Autodesk Inventor part; units mm, degrees
(part 6 of 7)
  line L1462 (-26.3463, 48.5084) -> (-12.9119, 48.5084)
  line L1463 (-12.9119, 52.5084) -> (-26.3463, 52.5084)
  line L1464 (-12.9119, 52.5084) -> (-26.3463, 52.5084)
  line L1465 (-26.3463, 48.5084) -> (-12.9119, 48.5084)
  line L1466 (-26.3463, 48.5084) -> (-12.9119, 48.5084)
  line L1467 (-26.3463, 48.5084) -> (-12.9119, 48.5084)
  arc A1650 (-12.9119, 48.5084) -> (-12.9119, 52.5084) centre (-12.9119, 50.5084) ccw
  arc A1651 (-46.3463, 52.5084) -> (-46.3463, 48.5084) centre (-46.3463, 50.5084) ccw
  arc A1652 (-52.9119, 48.5084) -> (-52.9119, 52.5084) centre (-52.9119, 50.5084) ccw
  arc A1653 (-46.3463, 52.5084) -> (-46.3463, 48.5084) centre (-46.3463, 50.5084) ccw
  arc A1654 (-46.3463, 52.5084) -> (-46.3463, 48.5084) centre (-46.3463, 50.5084) ccw
  arc A1655 (-46.3463, 52.5084) -> (-46.3463, 48.5084) centre (-46.3463, 50.5084) ccw
  arc A1656 (-46.3463, 52.5084) -> (-46.3463, 48.5084) centre (-46.3463, 50.5084) ccw
  arc A1657 (-46.3463, 52.5084) -> (-46.3463, 48.5084) centre (-46.3463, 50.5084) ccw
  arc A1658 (-52.9119, 48.5084) -> (-52.9119, 52.5084) centre (-52.9119, 50.5084) ccw
  arc A1659 (-52.9119, 48.5084) -> (-52.9119, 52.5084) centre (-52.9119, 50.5084) ccw
  arc A1660 (-52.9119, 48.5084) -> (-52.9119, 52.5084) centre (-52.9119, 50.5084) ccw
  arc A1661 (-52.9119, 48.5084) -> (-52.9119, 52.5084) centre (-52.9119, 50.5084) ccw
  line L1468 (-42.4124, 59.4654) -> (-55.8468, 59.4654)
  line L1469 (-55.8468, 55.4654) -> (-42.4124, 55.4654)
  line L1470 (-55.8468, 55.4654) -> (-42.4124, 55.4654)
  line L1471 (-55.8468, 55.4654) -> (-42.4124, 55.4654)
  line L1472 (-55.8468, 55.4654) -> (-42.4124, 55.4654)
  line L1473 (-55.8468, 55.4654) -> (-42.4124, 55.4654)
  line L1474 (-42.4124, 59.4654) -> (-55.8468, 59.4654)
  line L1475 (-42.4124, 59.4654) -> (-55.8468, 59.4654)
  line L1476 (-42.4124, 59.4654) -> (-55.8468, 59.4654)
  line L1477 (-42.4124, 59.4654) -> (-55.8468, 59.4654)
  arc A1662 (-86.3463, 52.5084) -> (-86.3463, 48.5084) centre (-86.3463, 50.5084) ccw
  arc A1663 (-86.3463, 52.5084) -> (-86.3463, 48.5084) centre (-86.3463, 50.5084) ccw
  arc A1664 (-86.3463, 52.5084) -> (-86.3463, 48.5084) centre (-86.3463, 50.5084) ccw
  arc A1665 (-92.9119, 48.5084) -> (-92.9119, 52.5084) centre (-92.9119, 50.5084) ccw
  line L1478 (-82.4124, 59.4654) -> (-95.8468, 59.4654)
  line L1479 (-95.8468, 55.4654) -> (-82.4124, 55.4654)
  line L1480 (-86.3463, 48.5084) -> (-72.9119, 48.5084)
  line L1481 (-86.3463, 48.5084) -> (-72.9119, 48.5084)
  line L1482 (-86.3463, 48.5084) -> (-72.9119, 48.5084)
  line L1483 (-72.9119, 52.5084) -> (-86.3463, 52.5084)
  line L1484 (-72.9119, 52.5084) -> (-86.3463, 52.5084)
  line L1485 (-72.9119, 52.5084) -> (-86.3463, 52.5084)
  arc A1666 (-75.8468, 59.4654) -> (-75.8468, 55.4654) centre (-75.8468, 57.4654) ccw
  arc A1667 (-75.8468, 59.4654) -> (-75.8468, 55.4654) centre (-75.8468, 57.4654) ccw
  arc A1668 (-75.8468, 59.4654) -> (-75.8468, 55.4654) centre (-75.8468, 57.4654) ccw
  arc A1669 (-75.8468, 59.4654) -> (-75.8468, 55.4654) centre (-75.8468, 57.4654) ccw
  arc A1670 (-82.4124, 55.4654) -> (-82.4124, 59.4654) centre (-82.4124, 57.4654) ccw
  line L1486 (-66.3463, 48.5084) -> (-52.9119, 48.5084)
  line L1487 (-52.9119, 52.5084) -> (-66.3463, 52.5084)
  line L1488 (-52.9119, 52.5084) -> (-66.3463, 52.5084)
  line L1489 (-66.3463, 48.5084) -> (-52.9119, 48.5084)
  line L1490 (-52.9119, 52.5084) -> (-66.3463, 52.5084)
  line L1491 (-52.9119, 52.5084) -> (-66.3463, 52.5084)
  line L1492 (-52.9119, 52.5084) -> (-66.3463, 52.5084)
  line L1493 (-66.3463, 48.5084) -> (-52.9119, 48.5084)
  line L1494 (-66.3463, 48.5084) -> (-52.9119, 48.5084)
  line L1495 (-66.3463, 48.5084) -> (-52.9119, 48.5084)
  line L1496 (-46.3463, 48.5084) -> (-32.9119, 48.5084)
  line L1497 (-32.9119, 52.5084) -> (-46.3463, 52.5084)
  line L1498 (-32.9119, 52.5084) -> (-46.3463, 52.5084)
  line L1499 (-46.3463, 48.5084) -> (-32.9119, 48.5084)
  line L1500 (-32.9119, 52.5084) -> (-46.3463, 52.5084)
  line L1501 (-32.9119, 52.5084) -> (-46.3463, 52.5084)
  line L1502 (-32.9119, 52.5084) -> (-46.3463, 52.5084)
  line L1503 (-46.3463, 48.5084) -> (-32.9119, 48.5084)
  line L1504 (-46.3463, 48.5084) -> (-32.9119, 48.5084)
  line L1505 (-46.3463, 48.5084) -> (-32.9119, 48.5084)
  line L1506 (-46.3463, 48.5084) -> (-32.9119, 48.5084)
  line L1507 (-32.9119, 52.5084) -> (-46.3463, 52.5084)
  arc A1671 (-55.8468, 59.4654) -> (-55.8468, 55.4654) centre (-55.8468, 57.4654) ccw
  arc A1672 (-55.8468, 59.4654) -> (-55.8468, 55.4654) centre (-55.8468, 57.4654) ccw
  arc A1673 (-55.8468, 59.4654) -> (-55.8468, 55.4654) centre (-55.8468, 57.4654) ccw
  arc A1674 (-62.4124, 55.4654) -> (-62.4124, 59.4654) centre (-62.4124, 57.4654) ccw
  arc A1675 (-55.8468, 59.4654) -> (-55.8468, 55.4654) centre (-55.8468, 57.4654) ccw
  arc A1676 (-55.8468, 59.4654) -> (-55.8468, 55.4654) centre (-55.8468, 57.4654) ccw
  arc A1677 (-55.8468, 59.4654) -> (-55.8468, 55.4654) centre (-55.8468, 57.4654) ccw
  arc A1678 (-55.8468, 59.4654) -> (-55.8468, 55.4654) centre (-55.8468, 57.4654) ccw
  arc A1679 (-62.4124, 55.4654) -> (-62.4124, 59.4654) centre (-62.4124, 57.4654) ccw
  arc A1680 (-62.4124, 55.4654) -> (-62.4124, 59.4654) centre (-62.4124, 57.4654) ccw
  arc A1681 (-66.3463, 52.5084) -> (-66.3463, 48.5084) centre (-66.3463, 50.5084) ccw
  arc A1682 (-72.9119, 48.5084) -> (-72.9119, 52.5084) centre (-72.9119, 50.5084) ccw
  arc A1683 (-66.3463, 52.5084) -> (-66.3463, 48.5084) centre (-66.3463, 50.5084) ccw
  line L1508 (-62.4124, 59.4654) -> (-75.8468, 59.4654)
  line L1509 (-75.8468, 55.4654) -> (-62.4124, 55.4654)
  arc A1684 (-72.9119, 48.5084) -> (-72.9119, 52.5084) centre (-72.9119, 50.5084) ccw
  line L1510 (-62.4124, 59.4654) -> (-75.8468, 59.4654)
  line L1511 (-75.8468, 55.4654) -> (-62.4124, 55.4654)
  arc A1685 (-66.3463, 52.5084) -> (-66.3463, 48.5084) centre (-66.3463, 50.5084) ccw
  arc A1686 (-66.3463, 52.5084) -> (-66.3463, 48.5084) centre (-66.3463, 50.5084) ccw
  arc A1687 (-66.3463, 52.5084) -> (-66.3463, 48.5084) centre (-66.3463, 50.5084) ccw
  line L1512 (-62.4124, 59.4654) -> (-75.8468, 59.4654)
  line L1513 (-75.8468, 55.4654) -> (-62.4124, 55.4654)
  arc A1688 (-72.9119, 48.5084) -> (-72.9119, 52.5084) centre (-72.9119, 50.5084) ccw
  arc A1689 (-106.3463, 52.5084) -> (-106.3463, 48.5084) centre (-106.3463, 50.5084) ccw
  arc A1690 (-95.8468, 59.4654) -> (-95.8468, 55.4654) centre (-95.8468, 57.4654) ccw
  line L1514 (-92.9119, 52.5084) -> (-106.3463, 52.5084)
  line L1515 (-106.3463, 48.5084) -> (-92.9119, 48.5084)
  arc A1691 (-35.8468, 59.4654) -> (-35.8468, 55.4654) centre (-35.8468, 57.4654) ccw
  arc A1692 (-35.8468, 59.4654) -> (-35.8468, 55.4654) centre (-35.8468, 57.4654) ccw
  arc A1693 (-35.8468, 59.4654) -> (-35.8468, 55.4654) centre (-35.8468, 57.4654) ccw
  arc A1694 (-42.4124, 55.4654) -> (-42.4124, 59.4654) centre (-42.4124, 57.4654) ccw
  arc A1695 (-42.4124, 55.4654) -> (-42.4124, 59.4654) centre (-42.4124, 57.4654) ccw
  arc A1696 (-35.8468, 59.4654) -> (-35.8468, 55.4654) centre (-35.8468, 57.4654) ccw
  arc A1697 (-35.8468, 59.4654) -> (-35.8468, 55.4654) centre (-35.8468, 57.4654) ccw
  arc A1698 (-35.8468, 59.4654) -> (-35.8468, 55.4654) centre (-35.8468, 57.4654) ccw
  arc A1699 (-35.8468, 59.4654) -> (-35.8468, 55.4654) centre (-35.8468, 57.4654) ccw
  arc A1700 (-35.8468, 59.4654) -> (-35.8468, 55.4654) centre (-35.8468, 57.4654) ccw
  arc A1701 (-35.8468, 59.4654) -> (-35.8468, 55.4654) centre (-35.8468, 57.4654) ccw
  arc A1702 (-42.4124, 55.4654) -> (-42.4124, 59.4654) centre (-42.4124, 57.4654) ccw
  arc A1703 (-42.4124, 55.4654) -> (-42.4124, 59.4654) centre (-42.4124, 57.4654) ccw
  arc A1704 (-42.4124, 55.4654) -> (-42.4124, 59.4654) centre (-42.4124, 57.4654) ccw
  arc A1705 (44.1532, 73.4654) -> (44.1532, 69.4654) centre (44.1532, 71.4654) ccw
  arc A1706 (44.1532, 73.4654) -> (44.1532, 69.4654) centre (44.1532, 71.4654) ccw
  arc A1707 (44.1532, 73.4654) -> (44.1532, 69.4654) centre (44.1532, 71.4654) ccw
  arc A1708 (44.1532, 73.4654) -> (44.1532, 69.4654) centre (44.1532, 71.4654) ccw
  arc A1709 (44.1532, 73.4654) -> (44.1532, 69.4654) centre (44.1532, 71.4654) ccw
  arc A1710 (44.1532, 73.4654) -> (44.1532, 69.4654) centre (44.1532, 71.4654) ccw
  arc A1711 (44.1532, 73.4654) -> (44.1532, 69.4654) centre (44.1532, 71.4654) ccw
  arc A1712 (33.6537, 66.5084) -> (33.6537, 62.5084) centre (33.6537, 64.5084) ccw
  arc A1713 (27.0881, 62.5084) -> (27.0881, 66.5084) centre (27.0881, 64.5084) ccw
  arc A1714 (27.0881, 62.5084) -> (27.0881, 66.5084) centre (27.0881, 64.5084) ccw
  arc A1715 (33.6537, 66.5084) -> (33.6537, 62.5084) centre (33.6537, 64.5084) ccw
  arc A1716 (27.0881, 62.5084) -> (27.0881, 66.5084) centre (27.0881, 64.5084) ccw
  arc A1717 (27.0881, 62.5084) -> (27.0881, 66.5084) centre (27.0881, 64.5084) ccw
  arc A1718 (27.0881, 62.5084) -> (27.0881, 66.5084) centre (27.0881, 64.5084) ccw
  arc A1719 (27.0881, 62.5084) -> (27.0881, 66.5084) centre (27.0881, 64.5084) ccw
  arc A1720 (33.6537, 66.5084) -> (33.6537, 62.5084) centre (33.6537, 64.5084) ccw
  arc A1721 (33.6537, 66.5084) -> (33.6537, 62.5084) centre (33.6537, 64.5084) ccw
  arc A1722 (33.6537, 66.5084) -> (33.6537, 62.5084) centre (33.6537, 64.5084) ccw
  line L1516 (24.1532, 69.4654) -> (37.5876, 69.4654)
  line L1517 (37.5876, 73.4654) -> (24.1532, 73.4654)
  line L1518 (24.1532, 69.4654) -> (37.5876, 69.4654)
  line L1519 (24.1532, 69.4654) -> (37.5876, 69.4654)
  line L1520 (24.1532, 69.4654) -> (37.5876, 69.4654)
  line L1521 (24.1532, 69.4654) -> (37.5876, 69.4654)
  line L1522 (24.1532, 69.4654) -> (37.5876, 69.4654)
  line L1523 (37.5876, 73.4654) -> (24.1532, 73.4654)
  line L1524 (37.5876, 73.4654) -> (24.1532, 73.4654)
  line L1525 (37.5876, 73.4654) -> (24.1532, 73.4654)
  line L1526 (37.5876, 73.4654) -> (24.1532, 73.4654)
  line L1527 (37.5876, 73.4654) -> (24.1532, 73.4654)
  arc A1723 (37.5876, 69.4654) -> (37.5876, 73.4654) centre (37.5876, 71.4654) ccw
  arc A1724 (37.5876, 69.4654) -> (37.5876, 73.4654) centre (37.5876, 71.4654) ccw
  arc A1725 (37.5876, 69.4654) -> (37.5876, 73.4654) centre (37.5876, 71.4654) ccw
  arc A1726 (37.5876, 69.4654) -> (37.5876, 73.4654) centre (37.5876, 71.4654) ccw
  arc A1727 (37.5876, 69.4654) -> (37.5876, 73.4654) centre (37.5876, 71.4654) ccw
  arc A1728 (37.5876, 69.4654) -> (37.5876, 73.4654) centre (37.5876, 71.4654) ccw
  arc A1729 (44.1532, 73.4654) -> (44.1532, 69.4654) centre (44.1532, 71.4654) ccw
  arc A1730 (47.0881, 62.5084) -> (47.0881, 66.5084) centre (47.0881, 64.5084) ccw
  arc A1731 (47.0881, 62.5084) -> (47.0881, 66.5084) centre (47.0881, 64.5084) ccw
  arc A1732 (53.6537, 66.5084) -> (53.6537, 62.5084) centre (53.6537, 64.5084) ccw
  arc A1733 (47.0881, 62.5084) -> (47.0881, 66.5084) centre (47.0881, 64.5084) ccw
  arc A1734 (47.0881, 62.5084) -> (47.0881, 66.5084) centre (47.0881, 64.5084) ccw
  arc A1735 (47.0881, 62.5084) -> (47.0881, 66.5084) centre (47.0881, 64.5084) ccw
  arc A1736 (53.6537, 66.5084) -> (53.6537, 62.5084) centre (53.6537, 64.5084) ccw
  arc A1737 (53.6537, 66.5084) -> (53.6537, 62.5084) centre (53.6537, 64.5084) ccw
  line L1528 (57.5876, 73.4654) -> (44.1532, 73.4654)
  line L1529 (44.1532, 69.4654) -> (57.5876, 69.4654)
  line L1530 (57.5876, 73.4654) -> (44.1532, 73.4654)
  line L1531 (44.1532, 69.4654) -> (57.5876, 69.4654)
  line L1532 (44.1532, 69.4654) -> (57.5876, 69.4654)
  line L1533 (44.1532, 69.4654) -> (57.5876, 69.4654)
  line L1534 (44.1532, 69.4654) -> (57.5876, 69.4654)
  line L1535 (57.5876, 73.4654) -> (44.1532, 73.4654)
  line L1536 (57.5876, 73.4654) -> (44.1532, 73.4654)
  line L1537 (57.5876, 73.4654) -> (44.1532, 73.4654)
  arc A1738 (57.5876, 69.4654) -> (57.5876, 73.4654) centre (57.5876, 71.4654) ccw
  arc A1739 (64.1532, 73.4654) -> (64.1532, 69.4654) centre (64.1532, 71.4654) ccw
  line L1538 (53.6537, 62.5084) -> (67.0881, 62.5084)
  line L1539 (53.6537, 62.5084) -> (67.0881, 62.5084)
  line L1540 (53.6537, 62.5084) -> (67.0881, 62.5084)
  line L1541 (67.0881, 66.5084) -> (53.6537, 66.5084)
  line L1542 (67.0881, 66.5084) -> (53.6537, 66.5084)
  line L1543 (67.0881, 66.5084) -> (53.6537, 66.5084)
  arc A1740 (64.1532, 73.4654) -> (64.1532, 69.4654) centre (64.1532, 71.4654) ccw
  arc A1741 (64.1532, 73.4654) -> (64.1532, 69.4654) centre (64.1532, 71.4654) ccw
  arc A1742 (64.1532, 73.4654) -> (64.1532, 69.4654) centre (64.1532, 71.4654) ccw
  arc A1743 (64.1532, 73.4654) -> (64.1532, 69.4654) centre (64.1532, 71.4654) ccw
  arc A1744 (57.5876, 69.4654) -> (57.5876, 73.4654) centre (57.5876, 71.4654) ccw
  arc A1745 (57.5876, 69.4654) -> (57.5876, 73.4654) centre (57.5876, 71.4654) ccw
  arc A1746 (57.5876, 69.4654) -> (57.5876, 73.4654) centre (57.5876, 71.4654) ccw
  arc A1747 (57.5876, 69.4654) -> (57.5876, 73.4654) centre (57.5876, 71.4654) ccw
  arc A1748 (67.0881, 62.5084) -> (67.0881, 66.5084) centre (67.0881, 64.5084) ccw
  arc A1749 (67.0881, 62.5084) -> (67.0881, 66.5084) centre (67.0881, 64.5084) ccw
  arc A1750 (67.0881, 62.5084) -> (67.0881, 66.5084) centre (67.0881, 64.5084) ccw
  line L1544 (77.5876, 73.4654) -> (64.1532, 73.4654)
  line L1545 (77.5876, 73.4654) -> (64.1532, 73.4654)
  line L1546 (77.5876, 73.4654) -> (64.1532, 73.4654)
  line L1547 (64.1532, 69.4654) -> (77.5876, 69.4654)
  line L1548 (64.1532, 69.4654) -> (77.5876, 69.4654)
  line L1549 (64.1532, 69.4654) -> (77.5876, 69.4654)
  arc A1751 (73.6537, 66.5084) -> (73.6537, 62.5084) centre (73.6537, 64.5084) ccw
  arc A1752 (77.5876, 69.4654) -> (77.5876, 73.4654) centre (77.5876, 71.4654) ccw
  arc A1753 (77.5876, 69.4654) -> (77.5876, 73.4654) centre (77.5876, 71.4654) ccw
  arc A1754 (77.5876, 69.4654) -> (77.5876, 73.4654) centre (77.5876, 71.4654) ccw
  arc A1755 (84.1532, 73.4654) -> (84.1532, 69.4654) centre (84.1532, 71.4654) ccw
  arc A1756 (84.1532, 73.4654) -> (84.1532, 69.4654) centre (84.1532, 71.4654) ccw
  line L1550 (87.0881, 66.5084) -> (73.6537, 66.5084)
  arc A1757 (87.0881, 62.5084) -> (87.0881, 66.5084) centre (87.0881, 64.5084) ccw
  line L1551 (73.6537, 62.5084) -> (87.0881, 62.5084)
  line L1552 (84.1532, 69.4654) -> (97.5876, 69.4654)
  line L1553 (97.5876, 73.4654) -> (84.1532, 73.4654)
  arc A1758 (97.5876, 69.4654) -> (97.5876, 73.4654) centre (97.5876, 71.4654) ccw
  line L1554 (33.6537, 62.5084) -> (47.0881, 62.5084)
  line L1555 (47.0881, 66.5084) -> (33.6537, 66.5084)
  line L1556 (33.6537, 62.5084) -> (47.0881, 62.5084)
  line L1557 (47.0881, 66.5084) -> (33.6537, 66.5084)
  line L1558 (47.0881, 66.5084) -> (33.6537, 66.5084)
  line L1559 (47.0881, 66.5084) -> (33.6537, 66.5084)
  line L1560 (47.0881, 66.5084) -> (33.6537, 66.5084)
  line L1561 (33.6537, 62.5084) -> (47.0881, 62.5084)
  line L1562 (33.6537, 62.5084) -> (47.0881, 62.5084)
  line L1563 (33.6537, 62.5084) -> (47.0881, 62.5084)
  arc A1759 (13.6537, 66.5084) -> (13.6537, 62.5084) centre (13.6537, 64.5084) ccw
  arc A1760 (13.6537, 66.5084) -> (13.6537, 62.5084) centre (13.6537, 64.5084) ccw
  arc A1761 (13.6537, 66.5084) -> (13.6537, 62.5084) centre (13.6537, 64.5084) ccw
  arc A1762 (13.6537, 66.5084) -> (13.6537, 62.5084) centre (13.6537, 64.5084) ccw
  arc A1763 (13.6537, 66.5084) -> (13.6537, 62.5084) centre (13.6537, 64.5084) ccw
  arc A1764 (13.6537, 66.5084) -> (13.6537, 62.5084) centre (13.6537, 64.5084) ccw
  arc A1765 (7.0881, 62.5084) -> (7.0881, 66.5084) centre (7.0881, 64.5084) ccw
  arc A1766 (7.0881, 62.5084) -> (7.0881, 66.5084) centre (7.0881, 64.5084) ccw
  arc A1767 (7.0881, 62.5084) -> (7.0881, 66.5084) centre (7.0881, 64.5084) ccw
  arc A1768 (7.0881, 62.5084) -> (7.0881, 66.5084) centre (7.0881, 64.5084) ccw
  arc A1769 (17.5876, 69.4654) -> (17.5876, 73.4654) centre (17.5876, 71.4654) ccw
  arc A1770 (17.5876, 69.4654) -> (17.5876, 73.4654) centre (17.5876, 71.4654) ccw
  arc A1771 (17.5876, 69.4654) -> (17.5876, 73.4654) centre (17.5876, 71.4654) ccw
  arc A1772 (17.5876, 69.4654) -> (17.5876, 73.4654) centre (17.5876, 71.4654) ccw
  arc A1773 (17.5876, 69.4654) -> (17.5876, 73.4654) centre (17.5876, 71.4654) ccw
  arc A1774 (17.5876, 69.4654) -> (17.5876, 73.4654) centre (17.5876, 71.4654) ccw
  arc A1775 (24.1532, 73.4654) -> (24.1532, 69.4654) centre (24.1532, 71.4654) ccw
  arc A1776 (24.1532, 73.4654) -> (24.1532, 69.4654) centre (24.1532, 71.4654) ccw
  arc A1777 (24.1532, 73.4654) -> (24.1532, 69.4654) centre (24.1532, 71.4654) ccw
  arc A1778 (24.1532, 73.4654) -> (24.1532, 69.4654) centre (24.1532, 71.4654) ccw
  arc A1779 (24.1532, 73.4654) -> (24.1532, 69.4654) centre (24.1532, 71.4654) ccw
  arc A1780 (24.1532, 73.4654) -> (24.1532, 69.4654) centre (24.1532, 71.4654) ccw
  arc A1781 (24.1532, 73.4654) -> (24.1532, 69.4654) centre (24.1532, 71.4654) ccw
  arc A1782 (24.1532, 73.4654) -> (24.1532, 69.4654) centre (24.1532, 71.4654) ccw
  arc A1783 (24.1532, 73.4654) -> (24.1532, 69.4654) centre (24.1532, 71.4654) ccw
  arc A1784 (4.1532, 73.4654) -> (4.1532, 69.4654) centre (4.1532, 71.4654) ccw
  arc A1785 (4.1532, 73.4654) -> (4.1532, 69.4654) centre (4.1532, 71.4654) ccw
  arc A1786 (4.1532, 73.4654) -> (4.1532, 69.4654) centre (4.1532, 71.4654) ccw
  arc A1787 (4.1532, 73.4654) -> (4.1532, 69.4654) centre (4.1532, 71.4654) ccw
  arc A1788 (4.1532, 73.4654) -> (4.1532, 69.4654) centre (4.1532, 71.4654) ccw
  arc A1789 (4.1532, 73.4654) -> (4.1532, 69.4654) centre (4.1532, 71.4654) ccw
  arc A1790 (4.1532, 73.4654) -> (4.1532, 69.4654) centre (4.1532, 71.4654) ccw
  arc A1791 (4.1532, 73.4654) -> (4.1532, 69.4654) centre (4.1532, 71.4654) ccw
  arc A1792 (4.1532, 73.4654) -> (4.1532, 69.4654) centre (4.1532, 71.4654) ccw
  arc A1793 (-2.4124, 69.4654) -> (-2.4124, 73.4654) centre (-2.4124, 71.4654) ccw
  arc A1794 (-2.4124, 69.4654) -> (-2.4124, 73.4654) centre (-2.4124, 71.4654) ccw
  arc A1795 (-2.4124, 69.4654) -> (-2.4124, 73.4654) centre (-2.4124, 71.4654) ccw
  arc A1796 (-2.4124, 69.4654) -> (-2.4124, 73.4654) centre (-2.4124, 71.4654) ccw
  arc A1797 (-32.9119, 62.5084) -> (-32.9119, 66.5084) centre (-32.9119, 64.5084) ccw
  arc A1798 (-32.9119, 62.5084) -> (-32.9119, 66.5084) centre (-32.9119, 64.5084) ccw
  arc A1799 (-32.9119, 62.5084) -> (-32.9119, 66.5084) centre (-32.9119, 64.5084) ccw
  arc A1800 (-32.9119, 62.5084) -> (-32.9119, 66.5084) centre (-32.9119, 64.5084) ccw
  arc A1801 (-32.9119, 62.5084) -> (-32.9119, 66.5084) centre (-32.9119, 64.5084) ccw
  arc A1802 (-32.9119, 62.5084) -> (-32.9119, 66.5084) centre (-32.9119, 64.5084) ccw
  line L1564 (27.0881, 66.5084) -> (13.6537, 66.5084)
  line L1565 (13.6537, 62.5084) -> (27.0881, 62.5084)
  line L1566 (27.0881, 66.5084) -> (13.6537, 66.5084)
  line L1567 (13.6537, 62.5084) -> (27.0881, 62.5084)
  line L1568 (13.6537, 62.5084) -> (27.0881, 62.5084)
  line L1569 (27.0881, 66.5084) -> (13.6537, 66.5084)
  line L1570 (27.0881, 66.5084) -> (13.6537, 66.5084)
  line L1571 (27.0881, 66.5084) -> (13.6537, 66.5084)
  line L1572 (13.6537, 62.5084) -> (27.0881, 62.5084)
  line L1573 (13.6537, 62.5084) -> (27.0881, 62.5084)
  line L1574 (13.6537, 62.5084) -> (27.0881, 62.5084)
  line L1575 (27.0881, 66.5084) -> (13.6537, 66.5084)
  line L1576 (4.1532, 69.4654) -> (17.5876, 69.4654)
  line L1577 (4.1532, 69.4654) -> (17.5876, 69.4654)
  line L1578 (4.1532, 69.4654) -> (17.5876, 69.4654)
  line L1579 (4.1532, 69.4654) -> (17.5876, 69.4654)
  line L1580 (4.1532, 69.4654) -> (17.5876, 69.4654)
  line L1581 (4.1532, 69.4654) -> (17.5876, 69.4654)
  line L1582 (17.5876, 73.4654) -> (4.1532, 73.4654)
  line L1583 (17.5876, 73.4654) -> (4.1532, 73.4654)
  line L1584 (17.5876, 73.4654) -> (4.1532, 73.4654)
  line L1585 (17.5876, 73.4654) -> (4.1532, 73.4654)
  line L1586 (17.5876, 73.4654) -> (4.1532, 73.4654)
  line L1587 (17.5876, 73.4654) -> (4.1532, 73.4654)
  arc A1803 (7.0881, 62.5084) -> (7.0881, 66.5084) centre (7.0881, 64.5084) ccw
  arc A1804 (7.0881, 62.5084) -> (7.0881, 66.5084) centre (7.0881, 64.5084) ccw
  line L1588 (-6.3463, 62.5084) -> (7.0881, 62.5084)
  line L1589 (7.0881, 66.5084) -> (-6.3463, 66.5084)
  line L1590 (7.0881, 66.5084) -> (-6.3463, 66.5084)
  line L1591 (-6.3463, 62.5084) -> (7.0881, 62.5084)
  line L1592 (-6.3463, 62.5084) -> (7.0881, 62.5084)
  line L1593 (7.0881, 66.5084) -> (-6.3463, 66.5084)
  line L1594 (7.0881, 66.5084) -> (-6.3463, 66.5084)
  line L1595 (7.0881, 66.5084) -> (-6.3463, 66.5084)
  line L1596 (-6.3463, 62.5084) -> (7.0881, 62.5084)
  line L1597 (-6.3463, 62.5084) -> (7.0881, 62.5084)
  line L1598 (-6.3463, 62.5084) -> (7.0881, 62.5084)
  line L1599 (7.0881, 66.5084) -> (-6.3463, 66.5084)
  arc A1805 (-6.3463, 66.5084) -> (-6.3463, 62.5084) centre (-6.3463, 64.5084) ccw
  arc A1806 (-6.3463, 66.5084) -> (-6.3463, 62.5084) centre (-6.3463, 64.5084) ccw
  arc A1807 (-6.3463, 66.5084) -> (-6.3463, 62.5084) centre (-6.3463, 64.5084) ccw
  arc A1808 (-6.3463, 66.5084) -> (-6.3463, 62.5084) centre (-6.3463, 64.5084) ccw
  arc A1809 (-6.3463, 66.5084) -> (-6.3463, 62.5084) centre (-6.3463, 64.5084) ccw
  arc A1810 (-6.3463, 66.5084) -> (-6.3463, 62.5084) centre (-6.3463, 64.5084) ccw
  arc A1811 (-12.9119, 62.5084) -> (-12.9119, 66.5084) centre (-12.9119, 64.5084) ccw
  arc A1812 (-12.9119, 62.5084) -> (-12.9119, 66.5084) centre (-12.9119, 64.5084) ccw
  arc A1813 (-12.9119, 62.5084) -> (-12.9119, 66.5084) centre (-12.9119, 64.5084) ccw
  arc A1814 (-12.9119, 62.5084) -> (-12.9119, 66.5084) centre (-12.9119, 64.5084) ccw
  arc A1815 (-12.9119, 62.5084) -> (-12.9119, 66.5084) centre (-12.9119, 64.5084) ccw
  line L1600 (-2.4124, 73.4654) -> (-15.8468, 73.4654)
  line L1601 (-15.8468, 69.4654) -> (-2.4124, 69.4654)
  line L1602 (-2.4124, 73.4654) -> (-15.8468, 73.4654)
  line L1603 (-15.8468, 69.4654) -> (-2.4124, 69.4654)
  line L1604 (-2.4124, 73.4654) -> (-15.8468, 73.4654)
  line L1605 (-15.8468, 69.4654) -> (-2.4124, 69.4654)
  line L1606 (-2.4124, 73.4654) -> (-15.8468, 73.4654)
  line L1607 (-15.8468, 69.4654) -> (-2.4124, 69.4654)
  line L1608 (-2.4124, 73.4654) -> (-15.8468, 73.4654)
  line L1609 (-15.8468, 69.4654) -> (-2.4124, 69.4654)
  line L1610 (-15.8468, 69.4654) -> (-2.4124, 69.4654)
  line L1611 (-2.4124, 73.4654) -> (-15.8468, 73.4654)
  arc A1816 (-2.4124, 69.4654) -> (-2.4124, 73.4654) centre (-2.4124, 71.4654) ccw
  arc A1817 (-2.4124, 69.4654) -> (-2.4124, 73.4654) centre (-2.4124, 71.4654) ccw
  arc A1818 (-15.8468, 73.4654) -> (-15.8468, 69.4654) centre (-15.8468, 71.4654) ccw
  arc A1819 (-15.8468, 73.4654) -> (-15.8468, 69.4654) centre (-15.8468, 71.4654) ccw
  arc A1820 (-15.8468, 73.4654) -> (-15.8468, 69.4654) centre (-15.8468, 71.4654) ccw
  arc A1821 (-15.8468, 73.4654) -> (-15.8468, 69.4654) centre (-15.8468, 71.4654) ccw
  arc A1822 (-15.8468, 73.4654) -> (-15.8468, 69.4654) centre (-15.8468, 71.4654) ccw
  arc A1823 (-22.4124, 69.4654) -> (-22.4124, 73.4654) centre (-22.4124, 71.4654) ccw
  arc A1824 (-22.4124, 69.4654) -> (-22.4124, 73.4654) centre (-22.4124, 71.4654) ccw
  arc A1825 (-15.8468, 73.4654) -> (-15.8468, 69.4654) centre (-15.8468, 71.4654) ccw
  arc A1826 (-15.8468, 73.4654) -> (-15.8468, 69.4654) centre (-15.8468, 71.4654) ccw
  arc A1827 (-22.4124, 69.4654) -> (-22.4124, 73.4654) centre (-22.4124, 71.4654) ccw
  arc A1828 (-15.8468, 73.4654) -> (-15.8468, 69.4654) centre (-15.8468, 71.4654) ccw
  arc A1829 (-15.8468, 73.4654) -> (-15.8468, 69.4654) centre (-15.8468, 71.4654) ccw
  arc A1830 (-22.4124, 69.4654) -> (-22.4124, 73.4654) centre (-22.4124, 71.4654) ccw
  arc A1831 (-22.4124, 69.4654) -> (-22.4124, 73.4654) centre (-22.4124, 71.4654) ccw
  arc A1832 (-22.4124, 69.4654) -> (-22.4124, 73.4654) centre (-22.4124, 71.4654) ccw
  arc A1833 (-26.3463, 66.5084) -> (-26.3463, 62.5084) centre (-26.3463, 64.5084) ccw
  arc A1834 (-26.3463, 66.5084) -> (-26.3463, 62.5084) centre (-26.3463, 64.5084) ccw
  arc A1835 (-26.3463, 66.5084) -> (-26.3463, 62.5084) centre (-26.3463, 64.5084) ccw
  arc A1836 (-26.3463, 66.5084) -> (-26.3463, 62.5084) centre (-26.3463, 64.5084) ccw
  arc A1837 (-26.3463, 66.5084) -> (-26.3463, 62.5084) centre (-26.3463, 64.5084) ccw
  arc A1838 (-26.3463, 66.5084) -> (-26.3463, 62.5084) centre (-26.3463, 64.5084) ccw
  line L1612 (-35.8468, 69.4654) -> (-22.4124, 69.4654)
  line L1613 (-35.8468, 69.4654) -> (-22.4124, 69.4654)
  line L1614 (-35.8468, 69.4654) -> (-22.4124, 69.4654)
  line L1615 (-35.8468, 69.4654) -> (-22.4124, 69.4654)
  line L1616 (-35.8468, 69.4654) -> (-22.4124, 69.4654)
  line L1617 (-35.8468, 69.4654) -> (-22.4124, 69.4654)
  line L1618 (-22.4124, 73.4654) -> (-35.8468, 73.4654)
  line L1619 (-22.4124, 73.4654) -> (-35.8468, 73.4654)
  line L1620 (-22.4124, 73.4654) -> (-35.8468, 73.4654)
  line L1621 (-22.4124, 73.4654) -> (-35.8468, 73.4654)
  line L1622 (-22.4124, 73.4654) -> (-35.8468, 73.4654)
  line L1623 (-22.4124, 73.4654) -> (-35.8468, 73.4654)
  line L1624 (-26.3463, 62.5084) -> (-12.9119, 62.5084)
  line L1625 (-12.9119, 66.5084) -> (-26.3463, 66.5084)
  line L1626 (-12.9119, 66.5084) -> (-26.3463, 66.5084)
  line L1627 (-26.3463, 62.5084) -> (-12.9119, 62.5084)
  line L1628 (-12.9119, 66.5084) -> (-26.3463, 66.5084)
  line L1629 (-12.9119, 66.5084) -> (-26.3463, 66.5084)
  line L1630 (-26.3463, 62.5084) -> (-12.9119, 62.5084)
  line L1631 (-12.9119, 66.5084) -> (-26.3463, 66.5084)
  line L1632 (-12.9119, 66.5084) -> (-26.3463, 66.5084)
  line L1633 (-26.3463, 62.5084) -> (-12.9119, 62.5084)
  line L1634 (-26.3463, 62.5084) -> (-12.9119, 62.5084)
  line L1635 (-26.3463, 62.5084) -> (-12.9119, 62.5084)
  arc A1839 (-12.9119, 62.5084) -> (-12.9119, 66.5084) centre (-12.9119, 64.5084) ccw
  arc A1840 (-46.3463, 66.5084) -> (-46.3463, 62.5084) centre (-46.3463, 64.5084) ccw
  arc A1841 (-52.9119, 62.5084) -> (-52.9119, 66.5084) centre (-52.9119, 64.5084) ccw
  arc A1842 (-46.3463, 66.5084) -> (-46.3463, 62.5084) centre (-46.3463, 64.5084) ccw
  arc A1843 (-46.3463, 66.5084) -> (-46.3463, 62.5084) centre (-46.3463, 64.5084) ccw
  arc A1844 (-46.3463, 66.5084) -> (-46.3463, 62.5084) centre (-46.3463, 64.5084) ccw
  arc A1845 (-46.3463, 66.5084) -> (-46.3463, 62.5084) centre (-46.3463, 64.5084) ccw
  arc A1846 (-46.3463, 66.5084) -> (-46.3463, 62.5084) centre (-46.3463, 64.5084) ccw
  arc A1847 (-52.9119, 62.5084) -> (-52.9119, 66.5084) centre (-52.9119, 64.5084) ccw
  arc A1848 (-52.9119, 62.5084) -> (-52.9119, 66.5084) centre (-52.9119, 64.5084) ccw
  arc A1849 (-52.9119, 62.5084) -> (-52.9119, 66.5084) centre (-52.9119, 64.5084) ccw
  arc A1850 (-52.9119, 62.5084) -> (-52.9119, 66.5084) centre (-52.9119, 64.5084) ccw
  line L1636 (-42.4124, 73.4654) -> (-55.8468, 73.4654)
  line L1637 (-55.8468, 69.4654) -> (-42.4124, 69.4654)
  line L1638 (-55.8468, 69.4654) -> (-42.4124, 69.4654)
  line L1639 (-55.8468, 69.4654) -> (-42.4124, 69.4654)
  line L1640 (-55.8468, 69.4654) -> (-42.4124, 69.4654)
  line L1641 (-55.8468, 69.4654) -> (-42.4124, 69.4654)
  line L1642 (-42.4124, 73.4654) -> (-55.8468, 73.4654)
  line L1643 (-42.4124, 73.4654) -> (-55.8468, 73.4654)
  line L1644 (-42.4124, 73.4654) -> (-55.8468, 73.4654)
  line L1645 (-42.4124, 73.4654) -> (-55.8468, 73.4654)
  arc A1851 (-86.3463, 66.5084) -> (-86.3463, 62.5084) centre (-86.3463, 64.5084) ccw
  arc A1852 (-86.3463, 66.5084) -> (-86.3463, 62.5084) centre (-86.3463, 64.5084) ccw
  arc A1853 (-86.3463, 66.5084) -> (-86.3463, 62.5084) centre (-86.3463, 64.5084) ccw
  arc A1854 (-92.9119, 62.5084) -> (-92.9119, 66.5084) centre (-92.9119, 64.5084) ccw
  line L1646 (-82.4124, 73.4654) -> (-95.8468, 73.4654)
  line L1647 (-95.8468, 69.4654) -> (-82.4124, 69.4654)
  line L1648 (-86.3463, 62.5084) -> (-72.9119, 62.5084)
  line L1649 (-86.3463, 62.5084) -> (-72.9119, 62.5084)
  line L1650 (-86.3463, 62.5084) -> (-72.9119, 62.5084)
  line L1651 (-72.9119, 66.5084) -> (-86.3463, 66.5084)
  line L1652 (-72.9119, 66.5084) -> (-86.3463, 66.5084)
  line L1653 (-72.9119, 66.5084) -> (-86.3463, 66.5084)
  arc A1855 (-75.8468, 73.4654) -> (-75.8468, 69.4654) centre (-75.8468, 71.4654) ccw
  arc A1856 (-75.8468, 73.4654) -> (-75.8468, 69.4654) centre (-75.8468, 71.4654) ccw
  arc A1857 (-75.8468, 73.4654) -> (-75.8468, 69.4654) centre (-75.8468, 71.4654) ccw
  arc A1858 (-75.8468, 73.4654) -> (-75.8468, 69.4654) centre (-75.8468, 71.4654) ccw
  arc A1859 (-82.4124, 69.4654) -> (-82.4124, 73.4654) centre (-82.4124, 71.4654) ccw
  line L1654 (-66.3463, 62.5084) -> (-52.9119, 62.5084)
  line L1655 (-52.9119, 66.5084) -> (-66.3463, 66.5084)
  line L1656 (-52.9119, 66.5084) -> (-66.3463, 66.5084)
  line L1657 (-66.3463, 62.5084) -> (-52.9119, 62.5084)
  line L1658 (-52.9119, 66.5084) -> (-66.3463, 66.5084)
  line L1659 (-52.9119, 66.5084) -> (-66.3463, 66.5084)
  line L1660 (-52.9119, 66.5084) -> (-66.3463, 66.5084)
  line L1661 (-66.3463, 62.5084) -> (-52.9119, 62.5084)
  line L1662 (-66.3463, 62.5084) -> (-52.9119, 62.5084)
  line L1663 (-66.3463, 62.5084) -> (-52.9119, 62.5084)
  line L1664 (-46.3463, 62.5084) -> (-32.9119, 62.5084)
  line L1665 (-32.9119, 66.5084) -> (-46.3463, 66.5084)
  line L1666 (-32.9119, 66.5084) -> (-46.3463, 66.5084)
  line L1667 (-46.3463, 62.5084) -> (-32.9119, 62.5084)
  line L1668 (-32.9119, 66.5084) -> (-46.3463, 66.5084)
  line L1669 (-32.9119, 66.5084) -> (-46.3463, 66.5084)
  line L1670 (-32.9119, 66.5084) -> (-46.3463, 66.5084)
  line L1671 (-46.3463, 62.5084) -> (-32.9119, 62.5084)
  line L1672 (-46.3463, 62.5084) -> (-32.9119, 62.5084)
  line L1673 (-46.3463, 62.5084) -> (-32.9119, 62.5084)
  line L1674 (-46.3463, 62.5084) -> (-32.9119, 62.5084)
  line L1675 (-32.9119, 66.5084) -> (-46.3463, 66.5084)
  arc A1860 (-55.8468, 73.4654) -> (-55.8468, 69.4654) centre (-55.8468, 71.4654) ccw
  arc A1861 (-55.8468, 73.4654) -> (-55.8468, 69.4654) centre (-55.8468, 71.4654) ccw
  arc A1862 (-55.8468, 73.4654) -> (-55.8468, 69.4654) centre (-55.8468, 71.4654) ccw
  arc A1863 (-62.4124, 69.4654) -> (-62.4124, 73.4654) centre (-62.4124, 71.4654) ccw
  arc A1864 (-55.8468, 73.4654) -> (-55.8468, 69.4654) centre (-55.8468, 71.4654) ccw
  arc A1865 (-55.8468, 73.4654) -> (-55.8468, 69.4654) centre (-55.8468, 71.4654) ccw
  arc A1866 (-55.8468, 73.4654) -> (-55.8468, 69.4654) centre (-55.8468, 71.4654) ccw
  arc A1867 (-55.8468, 73.4654) -> (-55.8468, 69.4654) centre (-55.8468, 71.4654) ccw
  arc A1868 (-62.4124, 69.4654) -> (-62.4124, 73.4654) centre (-62.4124, 71.4654) ccw
  arc A1869 (-62.4124, 69.4654) -> (-62.4124, 73.4654) centre (-62.4124, 71.4654) ccw
  arc A1870 (-66.3463, 66.5084) -> (-66.3463, 62.5084) centre (-66.3463, 64.5084) ccw
  arc A1871 (-72.9119, 62.5084) -> (-72.9119, 66.5084) centre (-72.9119, 64.5084) ccw
  arc A1872 (-66.3463, 66.5084) -> (-66.3463, 62.5084) centre (-66.3463, 64.5084) ccw
  line L1676 (-62.4124, 73.4654) -> (-75.8468, 73.4654)
  line L1677 (-75.8468, 69.4654) -> (-62.4124, 69.4654)
  arc A1873 (-72.9119, 62.5084) -> (-72.9119, 66.5084) centre (-72.9119, 64.5084) ccw
  line L1678 (-62.4124, 73.4654) -> (-75.8468, 73.4654)
  line L1679 (-75.8468, 69.4654) -> (-62.4124, 69.4654)
  arc A1874 (-66.3463, 66.5084) -> (-66.3463, 62.5084) centre (-66.3463, 64.5084) ccw
  arc A1875 (-66.3463, 66.5084) -> (-66.3463, 62.5084) centre (-66.3463, 64.5084) ccw
  arc A1876 (-66.3463, 66.5084) -> (-66.3463, 62.5084) centre (-66.3463, 64.5084) ccw
  line L1680 (-62.4124, 73.4654) -> (-75.8468, 73.4654)
  line L1681 (-75.8468, 69.4654) -> (-62.4124, 69.4654)
  arc A1877 (-72.9119, 62.5084) -> (-72.9119, 66.5084) centre (-72.9119, 64.5084) ccw
  arc A1878 (-106.3463, 66.5084) -> (-106.3463, 62.5084) centre (-106.3463, 64.5084) ccw
  arc A1879 (-95.8468, 73.4654) -> (-95.8468, 69.4654) centre (-95.8468, 71.4654) ccw
  line L1682 (-92.9119, 66.5084) -> (-106.3463, 66.5084)
  line L1683 (-106.3463, 62.5084) -> (-92.9119, 62.5084)
  arc A1880 (-35.8468, 73.4654) -> (-35.8468, 69.4654) centre (-35.8468, 71.4654) ccw
  arc A1881 (-35.8468, 73.4654) -> (-35.8468, 69.4654) centre (-35.8468, 71.4654) ccw
  arc A1882 (-35.8468, 73.4654) -> (-35.8468, 69.4654) centre (-35.8468, 71.4654) ccw
  arc A1883 (-42.4124, 69.4654) -> (-42.4124, 73.4654) centre (-42.4124, 71.4654) ccw
  arc A1884 (-42.4124, 69.4654) -> (-42.4124, 73.4654) centre (-42.4124, 71.4654) ccw
  arc A1885 (-35.8468, 73.4654) -> (-35.8468, 69.4654) centre (-35.8468, 71.4654) ccw
  arc A1886 (-35.8468, 73.4654) -> (-35.8468, 69.4654) centre (-35.8468, 71.4654) ccw
  arc A1887 (-35.8468, 73.4654) -> (-35.8468, 69.4654) centre (-35.8468, 71.4654) ccw
  arc A1888 (-35.8468, 73.4654) -> (-35.8468, 69.4654) centre (-35.8468, 71.4654) ccw
  arc A1889 (-35.8468, 73.4654) -> (-35.8468, 69.4654) centre (-35.8468, 71.4654) ccw
  arc A1890 (-35.8468, 73.4654) -> (-35.8468, 69.4654) centre (-35.8468, 71.4654) ccw
  arc A1891 (-42.4124, 69.4654) -> (-42.4124, 73.4654) centre (-42.4124, 71.4654) ccw
  arc A1892 (-42.4124, 69.4654) -> (-42.4124, 73.4654) centre (-42.4124, 71.4654) ccw
  arc A1893 (-42.4124, 69.4654) -> (-42.4124, 73.4654) centre (-42.4124, 71.4654) ccw
  line L1684 (-75, 70) -> (75, 70)
  line L1685 (85, 60) -> (85, -60)
  line L1686 (75, -70) -> (-75, -70)
  line L1687 (-85, -60) -> (-85, 60)
  line L1688 (85, 70) -> (-85, -70) construction
  line L1689 (-78, 73) -> (78, 73)
  line L1690 (88, 63) -> (88, -63)
  line L1691 (78, -73) -> (-78, -73)
  line L1692 (-88, -63) -> (-88, 63)
  line L1693 (-88, 73) -> (88, -73) construction
  arc A1894 (-75, 70) -> (-85, 60) centre (-75, 60) ccw
  arc A1895 (-78, 73) -> (-88, 63) centre (-78, 63) ccw
  arc A1896 (85, 60) -> (75, 70) centre (75, 60) ccw
  arc A1897 (88, 63) -> (78, 73) centre (78, 63) ccw
  arc A1898 (75, -70) -> (85, -60) centre (75, -60) ccw
  arc A1899 (78, -73) -> (88, -63) centre (78, -63) ccw
  arc A1900 (-88, -63) -> (-78, -73) centre (-78, -63) ccw
  arc A1901 (-85, -60) -> (-75, -70) centre (-75, -60) ccw
  circle A1902 centre (-73.7339, -61.8573) radius 1.25
  line L1694 (0, 0) -> (0, 1.4904)
  line L1695 (0, 0) -> (1.3651, 0)
  line L1696 (-73.7339, -52.8401) -> (-85, -52.8401)
  line L1697 (-64.7396, -62.5) -> (-64.7396, -70)
  arc A1903 (-64.7396, -62.5) -> (-74.5, -52.8727) centre (-73.7339, -61.8573) ccw
  arc A1904 (74.5, -52.8727) -> (64.7396, -62.5) centre (73.7339, -61.8573) ccw
  line L1698 (64.7396, -62.5) -> (64.7396, -70)
  line L1699 (73.7339, -52.8401) -> (85, -52.8401)
  circle A1905 centre (73.7339, -61.8573) radius 1.25
  line L1700 (-80, -42) -> (-77, -42)
  circle A1906 centre (-77, -42) radius 1.25
  arc A1907 (-69.0044, -42.2652) -> (-77, -34) centre (-77, -42) ccw
  line L1701 (-77, -34) -> (-85, -34)
  line L1702 (-69, -42) -> (-69, -54.1827)
  arc A1908 (77, -34) -> (69.0044, -42.2652) centre (77, -42) ccw
  line L1703 (69, -42) -> (69, -54.1827)
  circle A1909 centre (77, -42) radius 1.25
  line L1704 (-77, 34) -> (-85, 34)
  arc A1910 (-77, 34) -> (-69.0044, 42.2652) centre (-77, 42) ccw
  line L1705 (-69, 42) -> (-69, 54.1827)
  line L1706 (69, 42) -> (69, 54.1827)
  arc A1911 (69.0044, 42.2652) -> (77, 34) centre (77, 42) ccw
  line L1707 (77, -34) -> (85, -34)
  line L1708 (77, 34) -> (85, 34)
  line L1709 (64.7396, 62.5) -> (64.7396, 70)
  arc A1912 (64.7396, 62.5) -> (74.5, 52.8727) centre (73.7339, 61.8573) ccw
  line L1710 (73.7339, 52.8401) -> (85, 52.8401)
  circle A1913 centre (73.7339, 61.8573) radius 1.25
  line L1711 (-64.7396, 62.5) -> (-64.7396, 70)
  arc A1914 (-74.5, 52.8727) -> (-64.7396, 62.5) centre (-73.7339, 61.8573) ccw
  circle A1915 centre (-73.7339, 61.8573) radius 1.25
  line L1712 (-73.7339, 52.8401) -> (-85, 52.8401)
  circle A1916 centre (-73.7339, 61.8573) radius 1.25
  circle A1917 centre (73.7339, 61.8573) radius 1.25
  circle A1918 centre (77, 42) radius 1.25
  circle A1919 centre (-77, 42) radius 1.25
  point P0 (80, -38.5)
  point P1 (70, -38.5)
  point P2 (70, -48.5)
  point P3 (-70, -48.5)
  point P4 (-70, -38.5)
  point P5 (-80, -38.5)
  point P6 (80, -24.5)
  point P7 (70, -24.5)
  point P8 (70, -34.5)
  point P9 (-70, -34.5)
  point P10 (-70, -24.5)
  point P11 (-80, -24.5)
  point P12 (80, -10.5)
  point P13 (70, -10.5)
  point P14 (70, -20.5)
  point P15 (-70, -20.5)
  point P16 (-70, -10.5)
  point P17 (-80, -10.5)
  point P18 (80, 3.5)
  point P19 (70, 3.5)
  point P20 (70, -6.5)
  point P21 (-70, -6.5)
  point P22 (-70, 3.5)
  point P23 (-80, 3.5)
  point P24 (80, 17.5)
  point P25 (70, 17.5)
  point P26 (70, 7.5)
  point P27 (-70, 7.5)
  point P28 (-70, 17.5)
  point P29 (-80, 17.5)
  point P30 (80, 31.5)
  point P31 (70, 31.5)
  point P32 (70, 21.5)
  point P33 (-70, 21.5)
  point P34 (-70, 31.5)
  point P35 (-80, 31.5)
  point P36 (80, 45.5)
  point P37 (70, 45.5)
  point P38 (70, 35.5)
  point P39 (-70, 35.5)
  point P40 (-70, 45.5)
  point P41 (-80, 45.5)
  point P42 (80, 59.5)
  point P43 (70, 59.5)
  point P44 (70, 49.5)
  point P45 (-70, 49.5)
  point P46 (-70, 59.5)
  point P47 (-80, 59.5)
  point P48 (80, 73.5)
  point P49 (70, 73.5)
  point P50 (70, 63.5)
  point P51 (-70, 63.5)
  point P52 (-70, 73.5)
  point P53 (-80, 73.5)
  point P54 (80, -17.4916)
  point P55 (80, -7.4916)
  point P56 (80, -3.4916)
  point P57 (80, 6.5084)
  point P58 (80, 10.5084)
  point P59 (80, 20.5084)
  point P60 (80, 34)
  point P61 (74.1935, 34.5084)
  point P62 (71.7227, 35.9875)
  point P63 (69.0179, 41.4654)
  point P64 (69, 45.4654)
  point P65 (69, 49.9213)
  point P66 (69, 51.0956)
  point P67 (67.3736, 55.4654)
  point P68 (65.0397, 59.4654)
  point P69 (-65.0397, 59.4654)
  point P70 (-67.3736, 55.4654)
  point P71 (-69, 45.4654)
  point P72 (-69.0179, 41.4654)
  point P73 (-70.9314, 36.7873)
  point P74 (-74.1935, 34.5084)
  point P75 (-80, 34)
  point P76 (-80, 24.5084)
  point P77 (-80, 20.5084)
  point P78 (-80, 10.5084)
  point P79 (-80, 6.5084)
  point P80 (-80, -3.4916)
  point P81 (-80, -7.4916)
  point P82 (-80, -17.4916)
  point P83 (-80, -21.4916)
  point P84 (-80, -31.4916)
  point P85 (-72.4312, -35.433)
  point P86 (-69.7895, -38.5346)
  point P87 (-69, -42.5346)
  point P88 (-69, -52.5346)
  point P89 (-66.4553, -56.5346)
  point P90 (-65.0326, -59.4916)
  point P91 (-51.1847, -62.5)
  point P92 (-48.0735, -62.5)
  point P93 (-31.1847, -62.5)
  point P94 (-28.0735, -62.5)
  point P95 (-11.1847, -62.5)
  point P96 (-8.0735, -62.5)
  point P97 (8.8153, -62.5)
  point P98 (11.9265, -62.5)
  point P99 (28.8153, -62.5)
  point P100 (31.9265, -62.5)
  point P101 (48.8153, -62.5)
  point P102 (51.9265, -62.5)
  point P103 (65.0326, -59.4916)
  point P104 (66.4553, -56.5346)
  point P105 (69, -52.5346)
  point P106 (69, -48.0787)
  point P107 (69, -46.9044)
  point P108 (69, -42.5346)
  point P109 (69.7895, -38.5346)
  point P110 (72.7037, -35.2515)
  point P111 (80, -31.4916)
  point P112 (80, -21.4916)
  point P113 (-22.4124, 59.4654)
  point P114 (-2.4124, 59.4654)
  point P115 (-2.4124, 55.4654)
  point P116 (17.5876, 59.4654)
  point P117 (17.5876, 55.4654)
  point P118 (-22.4124, 45.4654)
  point P119 (-2.4124, 45.4654)
  point P120 (-2.4124, 41.4654)
  point P121 (17.5876, 45.4654)
  point P122 (17.5876, 41.4654)
  point P123 (44.1532, 41.4654)
  point P124 (44.1532, 27.4654)
  point P125 (53.6537, 10.5084)
  point P126 (44.1532, 13.4654)
  point P127 (53.6537, -3.4916)
  point P128 (44.1532, -0.5346)
  point P129 (53.6537, -17.4916)
  point P130 (44.1532, -14.5346)
  point P131 (64.1532, -28.5346)
  point P132 (-22.4124, -38.5346)
  point P133 (-2.4124, -38.5346)
  point P134 (-2.4124, -42.5346)
  point P135 (17.5876, -38.5346)
  point P136 (17.5876, -42.5346)
  point P137 (44.1532, -56.5346)
  point P138 (44.1532, -42.5346)
  point P139 (44.1532, -28.5346)
  point P140 (53.6537, -31.4916)
  point P141 (17.5876, -24.5346)
  point P142 (17.5876, -28.5346)
  point P143 (-2.4124, -24.5346)
  point P144 (-2.4124, -28.5346)
  point P145 (-22.4124, -24.5346)
  point P146 (-75.8468, -28.5346)
  point P147 (-75.8468, -24.5346)
  point P148 (64.1532, -14.5346)
  point P149 (17.5876, -10.5346)
  point P150 (17.5876, -14.5346)
  point P151 (-2.4124, -10.5346)
  point P152 (-2.4124, -14.5346)
  point P153 (-22.4124, -10.5346)
  point P154 (-75.8468, -14.5346)
  point P155 (-75.8468, -10.5346)
  point P156 (64.1532, -0.5346)
  point P157 (17.5876, 3.4654)
  point P158 (17.5876, -0.5346)
  point P159 (-2.4124, 3.4654)
  point P160 (-2.4124, -0.5346)
  point P161 (-22.4124, 3.4654)
  point P162 (-75.8468, -0.5346)
  point P163 (-75.8468, 3.4654)
  point P164 (64.1532, 13.4654)
  point P165 (17.5876, 17.4654)
  point P166 (17.5876, 13.4654)
  point P167 (-2.4124, 17.4654)
  point P168 (-2.4124, 13.4654)
  point P169 (-22.4124, 17.4654)
  point P170 (-75.8468, 13.4654)
  point P171 (-75.8468, 17.4654)
  point P172 (17.5876, 31.4654)
  point P173 (17.5876, 27.4654)
  point P174 (-2.4124, 31.4654)
  point P175 (-2.4124, 27.4654)
  point P176 (-22.4124, 31.4654)
  point P177 (-75.8468, 31.4654)
  point P178 (44.1532, 55.4654)
  dimension "d86" = 10
  dimension "d89" = 20
  dimension "d92" = 20
  dimension "d97" = 14
  dimension "d102" = 10
  dimension "d103" = 2.5
  dimension "d104" = 3
  dimension "d105" = 2.5
  constraints: 3829 point on circle, 3426 end point, 1920 centre point, 44 symmetric about line, 28 tangent, 11 point on line, 10 equal radius, 7 coincident, 6 horizontal, 6 parallel, 6 perpendicular, 3 vertical, 2 midpoint, 9473 other
  measures "d86" radius of A0
  measures "d89" distance of L6.end L16.end
  measures "d92" distance of L6.end L64.end
  measures "d97" distance of L6.start L220.start
  measures "d102" radius of A1894
  measures "d103" diameter of A1902
  measures "d104" distance of L1700.start L1700.end
  measures "d105" diameter of A1906
sketch "Esboço11" plane through (0, 0, 4) normal (0, 0, 1) x (1, 0, 0)
  line L0 (-75, 70) -> (75, 70)
  line L1 (85, 60) -> (85, -60)
  line L2 (75, -70) -> (-75, -70)
  line L3 (-85, -60) -> (-85, 60)
  line L4 (85, 70) -> (-85, -70) construction
  line L5 (-78, 73) -> (78, 73)
  line L6 (88, 63) -> (88, -63)
  line L7 (78, -73) -> (-78, -73)
  line L8 (-88, -63) -> (-88, 63)
  line L9 (-88, 73) -> (88, -73) construction
  arc A0 (-75, 70) -> (-85, 60) centre (-75, 60) ccw
  arc A1 (-78, 73) -> (-88, 63) centre (-78, 63) ccw
  arc A2 (85, 60) -> (75, 70) centre (75, 60) ccw
  arc A3 (88, 63) -> (78, 73) centre (78, 63) ccw
  arc A4 (75, -70) -> (85, -60) centre (75, -60) ccw
  arc A5 (78, -73) -> (88, -63) centre (78, -63) ccw
  arc A6 (-88, -63) -> (-78, -73) centre (-78, -63) ccw
  arc A7 (-85, -60) -> (-75, -70) centre (-75, -60) ccw
  circle A8 centre (-73.7339, -61.8573) radius 1.25
  line L10 (0, 0) -> (0, 1.4904)
  line L11 (0, 0) -> (1.3651, 0)
  line L12 (-73.7339, -52.8401) -> (-85, -52.8401)
  line L13 (-64.7396, -62.5) -> (-64.7396, -70)
  arc A9 (-64.7396, -62.5) -> (-74.5, -52.8727) centre (-73.7339, -61.8573) ccw
  arc A10 (74.5, -52.8727) -> (64.7396, -62.5) centre (73.7339, -61.8573) ccw
  line L14 (64.7396, -62.5) -> (64.7396, -70)
  line L15 (73.7339, -52.8401) -> (85, -52.8401)
  circle A11 centre (73.7339, -61.8573) radius 1.25
  line L16 (-80, -42) -> (-77, -42)
  circle A12 centre (-77, -42) radius 1.25
  arc A13 (-69.0044, -42.2652) -> (-77, -34) centre (-77, -42) ccw
  line L17 (-77, -34) -> (-85, -34)
  line L18 (-69, -42) -> (-69, -54.1827)
  arc A14 (77, -34) -> (69.0044, -42.2652) centre (77, -42) ccw
  line L19 (69, -42) -> (69, -54.1827)
  circle A15 centre (77, -42) radius 1.25
  line L20 (-77, 34) -> (-85, 34)
  arc A16 (-77, 34) -> (-69.0044, 42.2652) centre (-77, 42) ccw
  line L21 (-69, 42) -> (-69, 54.1827)
  line L22 (69, 42) -> (69, 54.1827)
  arc A17 (69.0044, 42.2652) -> (77, 34) centre (77, 42) ccw
  line L23 (77, -34) -> (85, -34)
  line L24 (77, 34) -> (85, 34)
  line L25 (64.7396, 62.5) -> (64.7396, 70)
  arc A18 (64.7396, 62.5) -> (74.5, 52.8727) centre (73.7339, 61.8573) ccw
  line L26 (73.7339, 52.8401) -> (85, 52.8401)
  circle A19 centre (73.7339, 61.8573) radius 1.25
  line L27 (-64.7396, 62.5) -> (-64.7396, 70)
  arc A20 (-74.5, 52.8727) -> (-64.7396, 62.5) centre (-73.7339, 61.8573) ccw
  circle A21 centre (-73.7339, 61.8573) radius 1.25
  line L28 (-73.7339, 52.8401) -> (-85, 52.8401)
  circle A22 centre (-73.7339, 61.8573) radius 1.25
  circle A23 centre (73.7339, 61.8573) radius 1.25
  circle A24 centre (77, 42) radius 1.25
  circle A25 centre (-77, 42) radius 1.25
  line L29 (70, -62.5) -> (-70, -62.5)
  line L30 (-80, -52.5) -> (-80, 52.5)
  line L31 (-70, 62.5) -> (70, 62.5)
  line L32 (80, 52.5) -> (80, -52.5)
  line L33 (80, -62.5) -> (-80, 62.5) construction
  line L34 (-80, -62.5) -> (80, 62.5) construction
  arc A26 (70, -62.5) -> (80, -52.5) centre (70, -52.5) ccw
  arc A27 (80, 52.5) -> (70, 62.5) centre (70, 52.5) ccw
  arc A28 (-70, 62.5) -> (-80, 52.5) centre (-70, 52.5) ccw
  arc A29 (-80, -52.5) -> (-70, -62.5) centre (-70, -52.5) ccw
  point P0 (80, -34)
  point P1 (80, 34)
  point P2 (-80, 34)
  point P3 (-80, -34)
  dimension "d106" = 10
  dimension "d107" = 2.5
  dimension "d108" = 3
  dimension "d109" = 2.5
  dimension "d110" = 160
  dimension "d111" = 125
  dimension "d112" = 10
  constraints: 70 end point, 49 point on circle, 44 symmetric about line, 30 centre point, 28 tangent, 19 point on line, 10 equal radius, 7 coincident, 6 parallel, 6 perpendicular, 4 horizontal, 4 midpoint, 2 vertical, 14 other
  measures "d106" radius of A0
  measures "d107" diameter of A8
  measures "d108" distance of L16.start L16.end
  measures "d109" diameter of A12
  measures "d110" distance of L33.end L34.end
  measures "d111" distance of L34.start L33.end
  measures "d112" radius of A26
extrude "Extrusão10" cut sketch "Esboço11" against normal blind 4 contours L31 A18 L22 A17 L24 L32 L23 A14 L19 A10 L29 A9 L18 A13 L17 L30 L20 A16 L21 A20
extrude "Extrusão11" add sketch "Esboço10" against normal blind 4 contours L0 A4 L4 A5 A6 L6 A7 A19 L16 A13 A28 L24 A22 A37 L32 A31 A46 L40 A1903 L50 A57 L49 L1702 L333 A351 L332 A1907 A548 L475 L1 L640 A737 L643 L808 A926 L811 L976 A1115 L979 L1144 A1304 L1147 L1704 A1910 L1312 A1493 L1341 A1485 L1340 L1705 A1914 L1509 A1674 L1508 L2 A1912 L1376 A1550 L1379 L1706 A1559 L1373 A1543 L1370 L1208 A1361 L1211 A1911 A1373 L1215 L1708 L3 L1046 A1184 L1047 L878 A995 L879 L710 A806 L711 L542 A617 L543 L374 A428 A1908 L200 A227 L203 L1703 A236 L197 A220 L194 L61 A69 L62 A1904 L60 A74 | L1215 A1373 A1911 | A1910 A1493 L1312
sketch "Esboço12" plane through (-80, 75, 4) normal (0, 1, 0) x (1, 0, 0)
  line L0 (3, 0) -> (0, 0) projected
  line L1 (0, 0) -> (0, 87)
  line L2 (0, 87) -> (160, 87)
  line L3 (0, 132) -> (0, 129)
  line L4 (0, 132) -> (3, 132) construction
  line L5 (0, 129) -> (160, 129)
  line L6 (0, 87) -> (0, 108)
  line L7 (0, 0) -> (0, 132) projected
  line L8 (0, 108) -> (26.67, 108)
  line L9 (26.67, 108) -> (53.34, 108)
  line L10 (53.34, 108) -> (80.01, 108)
  line L11 (80.01, 108) -> (106.68, 108)
  line L12 (106.68, 108) -> (133.35, 108)
  line L13 (133.35, 108) -> (160.02, 108)
  circle A0 centre (26.67, 108) radius 3.25
  circle A1 centre (53.34, 108) radius 3.75
  circle A2 centre (80.01, 108) radius 3.75
  circle A3 centre (106.68, 108) radius 3.75
  circle A4 centre (133.35, 108) radius 3.75
  point P0 (80, 4)
  dimension "d117" = 87
  dimension "d118" = 90
  dimension "d119" = 3
  dimension "d120" = 90
  dimension "d121" = 21
  dimension "d122" = 26.67
  dimension "d123" = 90
  dimension "d124" = 26.67
  dimension "d125" = 26.67
  dimension "d126" = 180
  dimension "d127" = 26.67
  dimension "d128" = 180
  dimension "d129" = 26.67
  dimension "d130" = 180
  dimension "d131" = 26.67
  dimension "d132" = 180
  dimension "d135" = 6.5
  dimension "d136" = 7.5
  dimension "d137" = 7.5
  dimension "d138" = 7.5
  dimension "d139" = 7.5
  constraints: 24 end point, 5 centre point, 5 coincident, 4 collinear, 2 perpendicular, 2 point on line, 1 horizontal
  measures "d117" distance of L0.end L1.end
  measures "d118" angle of L1 L2
  measures "d119" distance of L3.start L3.end
  measures "d120" angle of L3 L4
  measures "d121" distance of L1.end L6.end
  measures "d122" distance of L6.end L8.end
  measures "d123" angle of L6 L8
  measures "d124" distance of L8.end L9.end
  measures "d125" distance of L9.end L10.end
  measures "d126" angle of L10 L9
  measures "d127" distance of L10.end L11.end
  measures "d128" angle of L11 L10
  measures "d129" distance of L11.end L12.end
  measures "d130" angle of L12 L11
  measures "d131" distance of L12.end L13.end
  measures "d132" angle of L13 L12
  measures "d135" diameter of A0
  measures "d136" diameter of A1
  measures "d137" diameter of A2
  measures "d138" diameter of A3
  measures "d139" diameter of A4
extrude "Extrusão12" cut sketch "Esboço12" against normal blind 7
sketch "Esboço13" plane through (-80, 75, 4) normal (0, 1, 0) x (1, 0, 0)
  circle A0 centre (53.34, 108) radius 3.75 projected
  circle A1 centre (53.34, 108) radius 6.75
  circle A2 centre (80.01, 108) radius 3.75 projected
  circle A3 centre (80.01, 108) radius 6.75
  circle A4 centre (106.68, 108) radius 3.75 projected
  circle A5 centre (106.68, 108) radius 6.75
  circle A6 centre (133.35, 108) radius 3.75 projected
  circle A7 centre (133.35, 108) radius 6.75
  circle A8 centre (26.67, 108) radius 3.25 projected
  circle A9 centre (26.67, 108) radius 6
  point P0 (80, 4)
  dimension "d143" = 13.5
  dimension "d144" = 13.5
  dimension "d145" = 13.5
  dimension "d146" = 13.5
  dimension "d149" = 12
  constraints: 5 centre point, 5 coincident
  measures "d143" diameter of A1
  measures "d144" diameter of A3
  measures "d145" diameter of A5
  measures "d146" diameter of A7
  measures "d149" diameter of A9
extrude "Extrusão13" cut sketch "Esboço13" against normal blind 3